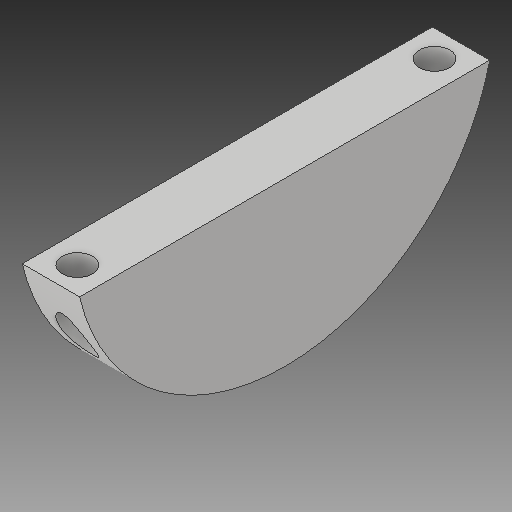
# Autodesk Inventor part: Contrapeso1
Saved by Autodesk Inventor 2019 (Build 230136000, 136)
## iProperties
Created: 2019-06-29
Part Number: Contrapeso1
Material: Generic
Document SubType Name: Modeling
Designer: usuario
Density: 1 g/cm^3
Appearance: Default
Mass: 6.16235 g
Surface Area: 27.8387 cm^2
Volume: 6.16235 cm^3
Author: usuario
Autodesk Inventor part; units mm, degrees
ref_plane "YZ Plane" through (0, 0, 0) normal (1, 0, 0) x (0, 1, 0)
ref_plane "XZ Plane" through (0, 0, 0) normal (0, 1, 0) x (-1, 0, 0)
ref_plane "XY Plane" through (0, 0, 0) normal (0, 0, 1) x (1, 0, 0)
sketch "Sketch1" plane through (0, 0, 0) normal (1, 0, 0) x (0, 1, 0)
  arc A0 (-1.2115, 27.4733) -> (-1.2115, -27.4733) centre (0, 0) ccw
  line L0 (-1.2115, -27.4733) -> (-6.2115, -27.4733)
  line L1 (-6.2115, -27.4733) -> (-6.2115, 27.4733)
  line L2 (-6.2115, 27.4733) -> (-1.2115, 27.4733)
  line L3 (-6.2115, -26.7893) -> (-6.2115, 26.7893)
  line L4 (-6.2115, 0) -> (-6.2115, 26.7893)
  circle A1 centre (0, 0) radius 27.5
  point P0 (5.2115, 24.6247)
  dimension "d0" = 5
  dimension "d1" = 53.5786
  constraints: 10 end point, 4 point on circle, 2 perpendicular, 2 point on line, 1 centre point, 1 coincident, 1 horizontal, 1 midpoint, 1 vertical, 3 other
  measures "d0" distance of L0.start L0.end
  measures "d1" distance of L3.end L3.start
extrude "Extrusion1" add sketch "Sketch1" along normal blind 7.5 contours L1 A0
sketch "Sketch2" plane through (0, -6.2115, 26.7893) normal (0, 1, 0) x (1, 0, 0)
  line L0 (0, 6.9167) -> (7.5, 6.9167)
  line L1 (0, 0) -> (0, 6.9167)
  line L2 (0, 6.9167) -> (7.5, 6.9167)
  line L3 (7.5, 26.7893) -> (7.5, 0)
  line L4 (7.5, 6.9167) -> (7.5, 0)
  line L5 (7.5, 0) -> (0, 0)
  line L6 (7.5, 0) -> (0, 0)
  circle A0 centre (3.75, 3.4583) radius 1
  line L7 (0, 0) -> (0, 53.5786)
  line L8 (0, 53.5786) -> (0, 0)
  line L9 (0, 26.7893) -> (7.5, 26.7893)
  circle A1 centre (3.75, 50.1203) radius 1
  circle A2 centre (3.75, 3.4583) radius 2
  circle A3 centre (3.75, 50.1203) radius 2
  line L10 (0, 6.9167) -> (7.5, 6.9167)
  line L11 (0, 0) -> (0, 6.9167)
  line L12 (0, 6.9167) -> (7.5, 6.9167)
  line L13 (7.5, 26.7893) -> (7.5, 0)
  line L14 (7.5, 6.9167) -> (7.5, 0)
  line L15 (7.5, 0) -> (0, 0)
  line L16 (7.5, 0) -> (0, 0)
  line L17 (0, 0) -> (2.2798, 2.1025)
  line L18 (5.2202, 4.8142) -> (7.5, 6.9167)
  line L19 (0, 6.9167) -> (2.2798, 4.8142)
  line L20 (5.2202, 2.1025) -> (7.5, 0)
  line L21 (0, 0) -> (0, 53.5786)
  line L22 (0, 53.5786) -> (0, 0)
  line L23 (0, 26.7893) -> (7.5, 26.7893)
  circle A4 centre (3.75, 50.1203) radius 1
  line L24 (0, 53.5786) -> (7.5, 53.5786)
  line L25 (7.5, 53.5786) -> (7.5, 0)
  circle A5 centre (3.75, 50.1203) radius 2
  circle A6 centre (3.75, 3.4583) radius 2
  point P0 (0, 26.7893)
  point P1 (280.32, 51.414)
  point P2 (4.4851, 4.1363)
  point P3 (4.4851, 2.7804)
  point P4 (3.0149, 4.1363)
  point P5 (3.0149, 2.7804)
  point P6 (280.32, 51.414)
  dimension "d6" = 2
  dimension "d9" = 4
  dimension "d10" = 4
  dimension "d13" = 4
  dimension "d14" = 4
  constraints: 52 end point, 8 point on circle, 7 centre point, 4 perpendicular, 4 vertical, 3 coincident, 3 collinear, 2 midpoint, 1 horizontal, 1 symmetric about line, 1 other
  measures "d6" diameter of A0
  measures "d9" diameter of A2
  measures "d10" diameter of A3
  measures "d13" diameter of A5
  measures "d14" diameter of A6
extrude "Extrusion2" cut sketch "Sketch2" against normal blind 10 contours A0 | A1
extrude "Extrusion3" cut sketch "Sketch2" against normal blind 13.175 contours A2 | A3
body "Solid1"
